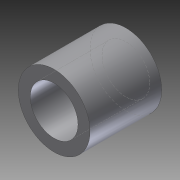
# Autodesk Inventor part: Kicker spacer
Saved by Autodesk Inventor 2012 (Build 160160000, 160)
## iProperties
Created: 2013-01-17
Part Number: Kicker spacer
Material: Default
Document SubType Name: Modeling
Designer: William
Density: 1 g/cm^3
Mass: 0.502749 g
Surface Area: 7.12557 cm^2
Volume: 0.502749 cm^3
Author: William
Autodesk Inventor part; units mm, degrees
ref_plane "YZ Plane" through (0, 0, 0) normal (1, 0, 0) x (0, 1, 0)
ref_plane "XZ Plane" through (0, 0, 0) normal (0, 1, 0) x (-1, 0, 0)
ref_plane "XY Plane" through (0, 0, 0) normal (0, 0, 1) x (1, 0, 0)
sketch "Sketch1" plane through (0, 0, 0) normal (0, 0, 1) x (1, 0, 0)
  circle A0 centre (-88.7279, 32.0599) radius 3.175
  circle A1 centre (-88.7279, 32.0599) radius 4.7625
  point P0 (0, 0)
  dimension "d0" = 6.35
  dimension "d2" = 9.525
  constraints: 2 centre point, 1 coincident
  measures "d0" diameter of A0
  measures "d2" diameter of A1
extrude "Extrusion1" add sketch "Sketch1" along normal blind 12.7
body "Solid1"
